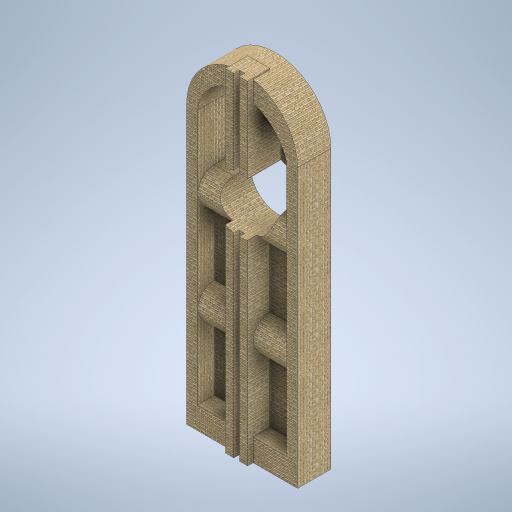
# Autodesk Inventor part: doorship
Saved by Autodesk Inventor 2023 (Build 270158000, 158)
## iProperties
Created: 2023-10-27
Part Number: doorship
Material: Wood (Oak)
Document SubType Name: Modeling
Designer: student
Density: 0.76 g/cm^3
Appearance: Plaid - Beige
Author: student
Autodesk Inventor part; units mm, degrees
ref_plane "YZ Plane" through (0, 0, 0) normal (1, 0, 0) x (0, 1, 0)
ref_plane "XZ Plane" through (0, 0, 0) normal (0, 1, 0) x (-1, 0, 0)
ref_plane "XY Plane" through (0, 0, 0) normal (0, 0, 1) x (1, 0, 0)
sketch "Sketch1" plane through (0, 0, 0) normal (0, 0, 1) x (1, 0, 0)
  line L0 (0, 0) -> (1000, 0)
  line L1 (1000, 0) -> (1000, 3000)
  line L2 (1000, 3000) -> (0, 3000)
  line L3 (0, 3000) -> (0, 0)
  dimension "d0" = 1000
  dimension "d1" = 3000
  constraints: 8 end point, 2 parallel, 1 horizontal, 1 perpendicular
  measures "d0" distance of L1.end L2.end
  measures "d1" distance of L0.end L1.end
extrude "Extrusion1" add sketch "Sketch1" along normal blind 250
fillet "Fillet1" radius 500 2 edges at (0, 3000, 125) (1000, 3000, 125)
sketch "Sketch2" plane through (1000, 0, 250) normal (1, 0, 0) x (0, 0, -1)
  line L0 (0, 0) -> (0, 2500) projected
  circle A0 centre (0, 950) radius 150
  circle A1 centre (0, 1850) radius 150
  line L1 (250, 0) -> (0, 0) projected
  line L2 (0, 2500) -> (250, 2500) projected
  point P0 (125, 2500)
  dimension "d5" = 300
  dimension "d6" = 300
  dimension "d7" = 950
  dimension "d8" = 900
  dimension "d9" = 650
  constraints: 2 centre point, 1 midpoint, 1 point on line
  measures "d5" diameter of A0
  measures "d6" diameter of A1
  measures "d7" distance from line of A0.centre L1
  measures "d8" distance of A1.centre A0.centre
  measures "d9" vertical distance of point (125, 2500) A1.centre
extrude "Extrusion2" add sketch "Sketch2" against normal blind 1000
sketch "Sketch3" plane through (0, 0, 0) normal (0, -1, 0) x (1, 0, 0)
  line L0 (1000, 250) -> (0, 250) projected
  line L1 (400, 250) -> (600, 250)
  line L2 (600, 250) -> (600, 450)
  line L3 (600, 450) -> (400, 450)
  line L4 (400, 450) -> (400, 250)
  line L5 (0, 0) -> (0, 250) projected
  dimension "d12" = 400
  dimension "d13" = 200
  dimension "d14" = 200
  constraints: 8 end point, 2 parallel, 1 horizontal, 1 perpendicular, 1 point on line
  measures "d12" distance between parallel lines of L5 L4
  measures "d13" distance of L2.end L3.end
  measures "d14" distance of L1.end L2.end
extrude "Extrusion3" add sketch "Sketch3" against normal blind 3000
sketch "Sketch4" plane through (0, 0, 250) normal (0, 0, 1) x (1, 0, 0)
  line L0 (600, 2989.8979) -> (600, 2000) projected
  line L1 (600, 2000) -> (600, 2989.8979)
  line L2 (600, 2000) -> (1000, 2000) projected
  line L3 (600, 2000) -> (1000, 2000)
  line L4 (1000, 2000) -> (1000, 2500) projected
  line L5 (1000, 2000) -> (1000, 2500)
  arc A0 (1000, 2500) -> (0, 2500) centre (500, 2500) ccw projected
  arc A1 (1000, 2500) -> (600, 2989.8979) centre (500, 2500) ccw
  point P0 (0, 0)
  constraints: 6 end point, 2 collinear, 2 point on circle, 1 centre point, 1 perpendicular
extrude "Extrusion4" cut sketch "Sketch4" against normal blind 100
sketch "Sketch5" plane through (0, 0, 250) normal (0, 0, 1) x (1, 0, 0)
  arc A0 (400, 2989.8979) -> (0, 2500) centre (500, 2500) ccw projected
  line L0 (400, 2989.8979) -> (400, 1992.9431)
  line L1 (400, 0) -> (400, 3000) projected
  line L2 (0, 2000) -> (400, 2000) projected
  line L3 (0, 2000) -> (0, 2500)
  arc A1 (500, 3000) -> (400, 2989.8979) centre (500, 2500) ccw projected
  arc A2 (400, 2989.8979) -> (0, 2500) centre (500, 2500) ccw
  point P0 (0, 0)
  constraints: 4 end point, 2 point on circle, 1 centre point, 1 point on line
extrude "Extrusion5" cut sketch "Sketch5" against normal blind 100
sketch "Sketch6" plane through (0, 0, 250) normal (0, 0, 1) x (1, 0, 0)
  line L0 (1000, 0) -> (1000, 2500) projected
  line L1 (600, 2000) -> (1000, 2000) projected
  line L2 (1000, 0) -> (900, 0)
  line L3 (900, 0) -> (900, 2000)
  line L4 (900, 2000) -> (1000, 2000)
  line L5 (1000, 2000) -> (1000, 0)
  point P0 (0, 0)
  point P1 (1000, 1250)
  dimension "d21" = 100
  constraints: 8 end point, 2 parallel, 1 horizontal, 1 midpoint, 1 perpendicular, 1 point on line
  measures "d21" distance from line of point (1000, 1250) L3
extrude "Extrusion6" add sketch "Sketch6" along normal blind 150
sketch "Sketch7" plane through (0, 0, 250) normal (0, 0, 1) x (1, 0, 0)
  line L0 (0, 2500) -> (0, 0) projected
  line L1 (0, 0) -> (400, 0) projected
  line L2 (0, 1993.85) -> (100, 1993.85)
  line L3 (100, 1993.85) -> (100, 0)
  line L4 (100, 0) -> (0, 0)
  line L5 (0, 0) -> (0, 1993.85)
  point P0 (0, 1250)
  dimension "d24" = 100
  constraints: 8 end point, 2 parallel, 2 point on line, 1 horizontal, 1 midpoint, 1 perpendicular
  measures "d24" distance from line of L3 point (0, 1250)
extrude "Extrusion7" add sketch "Sketch7" along normal blind 150
sketch "Sketch8" plane through (0, 0, 250) normal (0, 0, 1) x (1, 0, 0)
  line L0 (0, 1993.85) -> (0, 0) projected
  line L1 (1000, 0) -> (1000, 2000) projected
  line L2 (0, 0) -> (1000, 0)
  line L3 (1000, 0) -> (1000, 200)
  line L4 (1000, 200) -> (0, 200)
  line L5 (0, 200) -> (0, 0)
  line L6 (600, 0) -> (900, 0) projected
  point P0 (750, 0)
  point P1 (0, 200)
  dimension "d27" = 200
  constraints: 8 end point, 2 parallel, 1 horizontal, 1 midpoint, 1 perpendicular, 1 point on line
  measures "d27" distance from line of point (750, 0) L4
extrude "Extrusion8" add sketch "Sketch8" along normal blind 150
sketch "Sketch9" plane through (0, 0, 150) normal (0, 0, 1) x (1, 0, 0)
  arc A0 (1000, 2500) -> (0, 2500) centre (500, 2500) ccw projected
  line L0 (100, 1850) -> (100, 1993.85) projected
  line L1 (0, 2500) -> (100, 2500)
  line L2 (100, 2500) -> (100, 1993.85)
  line L3 (100, 1993.85) -> (0, 1993.85)
  line L4 (0, 1993.85) -> (0, 2500)
  line L5 (1000, 0) -> (1000, 2500) projected
  line L6 (900, 2000) -> (900, 1850) projected
  line L7 (1000, 2500) -> (900, 2500)
  line L8 (900, 2500) -> (900, 2000)
  line L9 (900, 2000) -> (1000, 2000)
  line L10 (1000, 2000) -> (1000, 2500)
  line L11 (600, 2000) -> (600, 2989.8979) projected
  arc A1 (600, 2810.0326) -> (100, 2500) centre (471.1061, 2459.7044) ccw
  line L12 (400, 2989.8979) -> (400, 2000) projected
  arc A2 (900, 2500) -> (400, 2826.1568) centre (455.7831, 2365.343) ccw
  point P0 (0, 0)
  point P1 (600, 2806.5489)
  constraints: 16 end point, 6 point on circle, 4 parallel, 2 centre point, 2 horizontal, 2 perpendicular, 2 point on line
extrude "Extrusion9" add sketch "Sketch9" along normal blind 250 contours L7 A2 L11 A0 | L5 L9 L8 L7 | L11 A1 L12 A0 | L12 A1 L1 A0 | L1 L2 L3 L4
sketch "Sketch10" plane through (0, 0, 0) normal (0, -1, 0) x (1, 0, 0)
  line L0 (400, 450) -> (600, 450) projected
  line L1 (475, 450) -> (525, 450)
  line L2 (525, 450) -> (525, 400)
  line L3 (525, 400) -> (475, 400)
  line L4 (475, 400) -> (475, 450)
  line L5 (400, 450) -> (400, 400) projected
  point P0 (0, 0)
  point P1 (525, 425)
  point P2 (475, 425)
  point P3 (500, 450)
  point P4 (500, 400)
  dimension "d32" = 50
  dimension "d33" = 50
  dimension "d34" = 75
  constraints: 8 end point, 4 midpoint, 2 parallel, 1 horizontal, 1 perpendicular, 1 point on line
  measures "d32" distance of point (525, 425) point (475, 425)
  measures "d33" distance of point (500, 450) point (500, 400)
  measures "d34" distance between parallel lines of L4 L5
extrude "Extrusion10" cut sketch "Sketch10" against normal blind 3000
sketch "Sketch11" plane through (0, 0, 0) normal (0, 0, -1) x (-1, 0, 0)
  line L0 (-525, 0) -> (-525, 3000) projected
  circle A0 centre (-525, 2000) radius 250
  line L1 (0, 0) -> (-1000, 0) projected
  dimension "d37" = 500
  dimension "d38" = 2000
  constraints: 1 centre point, 1 point on line
  measures "d37" diameter of A0
  measures "d38" distance from line of L1 A0.centre
extrude "Extrusion11" cut sketch "Sketch11" against normal blind 3000
sketch "Sketch12" plane through (0, 0, 0) normal (0, 0, -1) x (-1, 0, 0)
  line L0 (-1000, 0) -> (-1000, 2500) projected
  line L1 (0, 2500) -> (0, 0) projected
  line L2 (-1000, 0) -> (0, 0)
  line L3 (0, 0) -> (0, 2500)
  line L4 (0, 2500) -> (-1000, 2500)
  line L5 (-1000, 2500) -> (-1000, 0)
  line L6 (-525, 3000) -> (-525, 2250) projected
  arc A0 (0, 2500) -> (-1000, 2500) centre (-500, 2500.625) ccw
  constraints: 8 end point, 3 point on circle, 2 parallel, 1 centre point, 1 horizontal, 1 perpendicular
extrude "Extrusion12" [suppressed]
sketch "Sketch13" plane through (0, 0, 0) normal (0, 0, -1) x (-1, 0, 0)
  line L0 (-600, 0) -> (-1000, 0) projected
  arc A0 (0, 2500) -> (-400, 2989.8979) centre (-500, 2500) ccw projected
  line L1 (-1000, 0) -> (0, 0)
  line L2 (0, 0) -> (0, 2500)
  line L3 (0, 2500) -> (-1000, 2500)
  line L4 (-1000, 2500) -> (-1000, 0)
  circle A1 centre (-500, 2500) radius 500
  point P0 (0, 0)
  point P1 (-400, 2989.8979)
  constraints: 8 end point, 2 parallel, 1 coincident, 1 horizontal, 1 perpendicular, 3 other
extrude "Extrusion13" cut sketch "Sketch13" against normal blind 100
body "Solid1"
